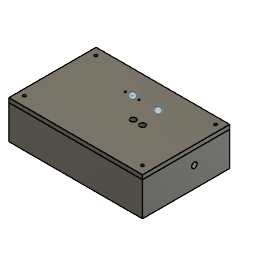
VehicleCase_v1 (Autodesk Fusion 360 design; units mm, degrees)
part number: 2026-06-20-03-10-33-368
part number: 2026-06-20-16-50-57-424
Autodesk Fusion 360 part; units mm, degrees
sketch "Sketch1" plane through (0, 0, 0) normal (0, 1, 0) x (1, 0, 0)
  line L0 (-73.8018, 46.4734) -> (73.8018, 46.4734)
  line L1 (73.8018, 46.4734) -> (73.8018, -46.4734)
  line L2 (73.8018, -46.4734) -> (-73.8018, -46.4734)
  line L3 (-73.8018, -46.4734) -> (-73.8018, 46.4734)
  line L4 (-73.8018, 46.4734) -> (73.8018, -46.4734) construction
  line L5 (73.8018, 46.4734) -> (-73.8018, -46.4734) construction
  constraint horizontal L0
  constraint perpendicular L0 L1
  constraint parallel L0 L2
  constraint parallel L1 L3
  constraint coincident L4 origin
  constraint coincident L5 origin
other "Base Mesh Feature1"
other "Modify1"
sketch "Sketch2" plane through (0, 0, 0) normal (0, 1, 0) x (1, 0, 0)
  line L0 (78.8018, -51.4734) -> (-78.8018, -51.4734)
  line L1 (-78.8018, -51.4734) -> (-78.8018, 51.4734)
  line L2 (-78.8018, 51.4734) -> (78.8018, 51.4734)
  line L3 (78.8018, 51.4734) -> (78.8018, -51.4734)
  line L4 (78.8018, -51.4734) -> (-78.8018, 51.4734) construction
  line L5 (-78.8018, -51.4734) -> (78.8018, 51.4734) construction
  line L6 (-73.8018, -46.4734) -> (-73.8018, 46.4734)
  line L7 (-73.8018, 46.4734) -> (73.8018, 46.4734)
  line L8 (73.8018, 46.4734) -> (73.8018, -46.4734)
  line L9 (73.8018, -46.4734) -> (-73.8018, -46.4734)
  dimension "d1" = 5
  dimension "d2" = 5
  dimension "d3" = 5
  dimension "d4" = 5
  constraint horizontal L0
  constraint perpendicular L0 L1
  constraint parallel L0 L2
  constraint parallel L1 L3
  constraint coincident L4 origin
  constraint coincident L5 origin
  measures "d1" distance of L1 L6
  measures "d2" distance of L2 L7
  measures "d3" distance of L3 L8
  measures "d4" distance of L0 L9
extrude "Extrude1" add sketch "Sketch2" along normal blind 40 makes body 1
extrude "Extrude2" add sketch "Sketch1" along normal blind 5 bodies 1
other "Modify2"
other "Modify3"
other "Modify4"
other "Modify5"
other "Modify6"
other "Modify7"
sketch "Sketch3" plane through (0, 5, 0) normal (0, 1, 0) x (-1, 0, 0)
  line L0 (73.8018, 46.4734) -> (-73.8018, 46.4734)
  line L1 (-73.8018, 46.4734) -> (-73.8018, -46.4734)
  line L2 (-73.8018, -46.4734) -> (73.8018, -46.4734)
  line L3 (73.8018, -46.4734) -> (73.8018, 46.4734)
  circle A0 centre (-50.0252, 26.8886) radius 4
  circle A1 centre (42.999, 26.8866) radius 4
  circle A2 centre (42.967, -26.1006) radius 4
  circle A3 centre (-49.0372, -26.0946) radius 4
  circle A4 centre (-50.0252, 26.8886) radius 2.8
  circle A5 centre (42.999, 26.8866) radius 2.8
  circle A6 centre (42.967, -26.1006) radius 2.8
  circle A7 centre (-49.0372, -26.0946) radius 2.8
  dimension "d9" = 8
  dimension "d10" = 8
  dimension "d11" = 8
  dimension "d12" = 8
  dimension "d13" = 5.6
  dimension "d14" = 5.6
  dimension "d15" = 5.6
  dimension "d16" = 5.6
  constraint concentric A0 A4
  constraint concentric A1 A5
  constraint concentric A2 A6
  constraint concentric A3 A7
  measures "d9" diameter of A0
  measures "d10" diameter of A1
  measures "d11" diameter of A2
  measures "d12" diameter of A3
  measures "d13" diameter of A4
  measures "d14" diameter of A5
  measures "d15" diameter of A6
  measures "d16" diameter of A7
extrude "Extrude3" add sketch "Sketch3" along normal blind 20 contours A0 bodies 1
extrude "Extrude4" add 1 faces at (51.6323, 5, 27.6626) along direction (0, 1, 0) blind 30 on bodies 1 bodies 1
extrude "Extrude5" add sketch "Sketch3" along normal blind 20 contours A1 bodies 1
extrude "Extrude6" add sketch "Sketch3" along normal blind 30 contours A5 bodies 1
extrude "Extrude7" add sketch "Sketch3" along normal blind 20 contours A2 bodies 1
extrude "Extrude8" add sketch "Sketch3" along normal blind 30 contours A6 bodies 1
extrude "Extrude9" add sketch "Sketch3" along normal blind 20 contours A3 bodies 1
extrude "Extrude10" add sketch "Sketch3" along normal blind 30 contours A7 bodies 1
other "Modify8"
other "Modify9"
copy_body "Body->Comp1" bodies 1 removing the originals makes body 2 in component "Component"
other "Modify10"
other "Modify11"
other "Modify12"
sketch "Sketch4" plane through (0, 0, 0) normal (0, 1, 0) x (1, 0, 0)
  line L0 (-39.9998, 12.764) -> (40.0002, 12.764)
  line L1 (40.0002, 12.764) -> (40.0002, -10.236)
  line L2 (40.0002, -10.236) -> (-39.9998, -10.236)
  line L3 (-39.9998, -10.236) -> (-39.9998, 12.764)
  line L4 (-73.8018, 46.4734) -> (-73.8018, -46.4734)
  line L5 (73.8018, -46.4734) -> (73.8018, 46.4734)
  dimension "d37" = 80
  dimension "d38" = 23
  dimension "d39" = 33.802
  dimension "d40" = 33.8017
  constraint horizontal L0
  constraint vertical L1
  constraint horizontal L2
  constraint vertical L3
  measures "d37" distance of L0.start L0.end
  measures "d38" distance of L0.start L2.end
  measures "d39" distance of L3 L4
  measures "d40" distance of L1 L5
extrude "Extrude2'" cut sketch "Sketch4" along normal blind 21 bodies 2 in component "Component"
chamfer "Chamfer1" distance 20 angle 45 1 edges at (-73.8018, 22.5, -46.4734) on bodies 2 in component "Component"
chamfer "Chamfer2" distance 20 angle 45 1 edges at (-73.8018, 22.5, 46.4734) on bodies 2 in component "Component"
chamfer "Chamfer3" distance 20 angle 45 1 edges at (73.8018, 22.5, 46.4734) on bodies 2 in component "Component"
chamfer "Chamfer4" distance 20 angle 45 1 edges at (73.8018, 22.5, -46.4734) on bodies 2 in component "Component"
hole "Hole1" at (-78.8018, 24.1985, -9.5796) direction (1, 0, 0) diameter 6.5 depth 15 tip angle 118 bodies 2 in component "Component"
hole "Hole2" at (78.8018, 24.1475, -9.7743) direction (-1, 0, 0) diameter 6.5 depth 15 tip angle 118 bodies 2 in component "Component"
sketch "Sketch6" plane through (73.8018, 0, 0) normal (-1, 0, 0) x (0, 0, 1)
  circle A0 centre (-9.7743, 24.1475) radius 3.25
  line L0 (-26.4734, 40) -> (-26.4734, 5)
  line L1 (-26.4734, 5) -> (26.4734, 5)
  line L2 (26.4734, 5) -> (26.4734, 40)
  line L3 (26.4734, 40) -> (-26.4734, 40)
sketch "Sketch7" plane through (0, 0, 0) normal (0, 1, 0) x (1, 0, 0)
  line L0 (-44.9998, 17.764) -> (45.0002, 17.764)
  line L1 (45.0002, 17.764) -> (45.0002, -15.236)
  line L2 (45.0002, -15.236) -> (-44.9998, -15.236)
  line L3 (-44.9998, -15.236) -> (-44.9998, 17.764)
  line L4 (40.0002, 12.764) -> (40.0002, -10.236)
  line L5 (-39.9998, 12.764) -> (40.0002, 12.764)
  line L6 (-39.9998, -10.236) -> (-39.9998, 12.764)
  line L7 (40.0002, -10.236) -> (-39.9998, -10.236)
  dimension "d53" = 5
  dimension "d54" = 5
  dimension "d55" = 5
  dimension "d56" = 5
  constraint horizontal L0
  constraint vertical L1
  constraint horizontal L2
  constraint vertical L3
  measures "d53" distance of L1 L4
  measures "d54" distance of L0 L5
  measures "d55" distance of L3 L6
  measures "d56" distance of L2 L7
extrude "Extrude3'" add sketch "Sketch7" along normal blind 21 contours L0 L1 L2 L3 | L4 L5 L6 L7 bodies 2 in component "Component"
extrude "Extrude4'" cut sketch "Sketch4" along normal blind 25 bodies 2 in component "Component"
other "Modify13"
other "Modify14"
hole "Hole3" at (1.2176, 21.7353, -51.4734) direction (0, 0, 1) diameter 6.5 depth 15 tip angle 118 bodies 2 in component "Component"
other "Modify15"
sketch "Sketch8" plane through (0, 40, 0) normal (0, 1, 0) x (-1, 0, 0)
  line L0 (-73.8018, -26.4734) -> (-73.8018, 26.4734)
  line L1 (-73.8018, 26.4734) -> (-53.8018, 46.4734)
  line L2 (-53.8018, 46.4734) -> (53.8018, 46.4734)
  line L3 (53.8018, 46.4734) -> (73.8018, 26.4734)
  line L4 (73.8018, 26.4734) -> (73.8018, -26.4734)
  line L5 (73.8018, -26.4734) -> (53.8018, -46.4734)
  line L6 (53.8018, -46.4734) -> (-53.8018, -46.4734)
  line L7 (-53.8018, -46.4734) -> (-73.8018, -26.4734)
  line L8 (-78.8018, -51.4734) -> (78.8018, -51.4734)
  line L9 (78.8018, -51.4734) -> (78.8018, 51.4734)
  line L10 (78.8018, 51.4734) -> (-78.8018, 51.4734)
  line L11 (-78.8018, 51.4734) -> (-78.8018, -51.4734)
  line L12 (78.8018, -51.4734) -> (-78.8018, -51.4734)
  line L13 (-78.8018, -51.4734) -> (-78.8018, 51.4734)
  line L14 (-78.8018, 51.4734) -> (78.8018, 51.4734)
  line L15 (78.8018, 51.4734) -> (78.8018, -51.4734)
  constraint horizontal L12
  constraint vertical L13
  constraint horizontal L14
  constraint vertical L15
  constraint coincident L10.end L11.start
  constraint coincident L8.end L9.start
extrude "Extrude5'" add sketch "Sketch8" along normal blind 5 separate body contours L0 L1 L2 L3 L4 L5 L6 L7 | L8 L9 L10 L11 L12 L13 L14 L15 makes body 3 in component "Component"
hole "Hole4" at (17.0576, 45, 0.5249) direction (0, -1, 0) diameter 6.5 depth 15 tip angle 118 bodies 3 in component "Component"
hole "Hole5" at (28.1632, 45, 0.6139) direction (0, -1, 0) diameter 6.5 depth 15 tip angle 118 bodies 3 in component "Component"
hole "Hole6" at (-15.9923, 45, -23.2284) direction (0, -1, 0) diameter 2 depth 15 tip angle 118 bodies 3 in component "Component"
hole "Hole7" at (-7.9177, 45, -23.2781) direction (0, -1, 0) diameter 2 depth 15 tip angle 118 bodies 3 in component "Component"
hole "Hole8" at (0.1073, 45, -23.1539) direction (0, -1, 0) diameter 2 depth 15 tip angle 118 bodies 3 in component "Component"
sketch "Sketch9" plane through (0, 0, 0) normal (0, 1, 0) x (1, 0, 0)
  circle A0 centre (-52.8021, 68.5609) radius 3.5
  circle A1 centre (-22.8021, 68.5609) radius 3.5
  circle A2 centre (-52.8021, 68.5609) radius 2.75
  circle A3 centre (-22.8021, 68.5609) radius 2.75
  dimension "d81" = 7
  dimension "d82" = 7
  dimension "d83" = 5.5
  dimension "d84" = 5.5
  constraint concentric A0 A2
  constraint concentric A1 A3
  measures "d81" diameter of A0
  measures "d82" diameter of A1
  measures "d83" diameter of A2
  measures "d84" diameter of A3
extrude "Extrude11" add sketch "Sketch9" along normal blind 3 separate body contours A0 makes body 4
extrude "Extrude12" add sketch "Sketch9" along normal blind 10 contours A2 bodies 4
extrude "Extrude13" add sketch "Sketch9" along normal blind 3 separate body contours A1 makes body 5
extrude "Extrude14" add sketch "Sketch9" along normal blind 10 contours A3 bodies 5
other "Modify16"
hole "Hole9" at (-70.4475, 40, -42.7802) direction (0, -1, 0) diameter 2.8 depth 15 tip angle 118 bodies 2 in component "Component"
hole "Hole10" at (70.4371, 40, -43.0376) direction (0, -1, 0) diameter 2.8 depth 15 tip angle 118 bodies 2 in component "Component"
hole "Hole11" at (-71.5455, 40, 40.3184) direction (0, -1, 0) diameter 2.8 depth 15 tip angle 118 bodies 2 in component "Component"
hole "Hole12" at (69.1628, 40, 41.8331) direction (0, -1, 0) diameter 2.8 depth 15 tip angle 118 bodies 2 in component "Component"
hole "Hole13" at (-70.4536, 45, -42.7966) direction (0, -1, 0) diameter 3.2 depth 5 tip angle 118 bodies 2 3 in component "Component"
hole "Hole14" at (70.4418, 45, -43.0281) direction (0, -1, 0) diameter 3.2 depth 5 tip angle 118 bodies 2 3 in component "Component"
hole "Hole15" at (-71.5432, 45, 40.3174) direction (0, -1, 0) diameter 3.2 depth 5 tip angle 118 bodies 2 3 in component "Component"
hole "Hole16" at (69.1625, 45, 41.8306) direction (0, -1, 0) diameter 3.2 depth 5 tip angle 118 bodies 2 3 in component "Component"
fillet "Fillet1" radius 2 1 faces at (-50.2681, 5.3333, -67.4927) on bodies 4
fillet "Fillet2" radius 2 1 edges at (-25.366, 10, -67.5665) 1 faces at (-20.1372, 7.6667, -67.8823) on bodies 5
component "Component" placed x (1, 0, 0) y (0, 1, 0) z (0, 0, 1) at (0, 0, 0)
